Autodesk Inventor part; units mm, degrees
(part 2 of 2)
  line L767 (227.5411, -183.5124) -> (230.4279, -188.5124)
  line L768 (221.7676, -183.5124) -> (227.5411, -183.5124)
  line L769 (221.7676, -208.5124) -> (218.8809, -203.5124)
  line L770 (218.8809, -203.5124) -> (221.7676, -198.5124)
  line L771 (221.7676, -193.5124) -> (218.8809, -188.5124)
  line L772 (218.8809, -188.5124) -> (221.7676, -183.5124)
  line L773 (217.4375, -211.0124) -> (214.5507, -216.0124)
  line L774 (214.5507, -221.0124) -> (217.4375, -226.0124)
  line L775 (217.4375, -226.0124) -> (214.5507, -231.0124)
  line L776 (208.7772, -221.0124) -> (214.5507, -221.0124)
  line L777 (214.5507, -231.0124) -> (208.7772, -231.0124)
  line L778 (208.7772, -231.0124) -> (205.8905, -226.0124)
  line L779 (205.8905, -226.0124) -> (208.7772, -221.0124)
  line L780 (214.5507, -206.0124) -> (217.4375, -211.0124)
  line L781 (214.5507, -216.0124) -> (208.7772, -216.0124)
  line L782 (208.7772, -216.0124) -> (205.8905, -211.0124)
  line L783 (208.7772, -206.0124) -> (214.5507, -206.0124)
  line L784 (205.8905, -211.0124) -> (208.7772, -206.0124)
  line L785 (218.8809, -218.5124) -> (221.7676, -213.5124)
  line L786 (221.7676, -213.5124) -> (227.5411, -213.5124)
  line L787 (227.5411, -213.5124) -> (230.4279, -218.5124)
  line L788 (227.5411, -223.5124) -> (221.7676, -223.5124)
  line L789 (230.4279, -218.5124) -> (227.5411, -223.5124)
  line L790 (221.7676, -223.5124) -> (218.8809, -218.5124)
  line L791 (217.4375, -181.0124) -> (214.5507, -186.0124)
  line L792 (208.7772, -186.0124) -> (205.8905, -181.0124)
  line L793 (214.5507, -186.0124) -> (208.7772, -186.0124)
  line L794 (214.5507, -191.0124) -> (217.4375, -196.0124)
  line L795 (205.8905, -196.0124) -> (208.7772, -191.0124)
  line L796 (217.4375, -196.0124) -> (214.5507, -201.0124)
  line L797 (208.7772, -201.0124) -> (205.8905, -196.0124)
  line L798 (214.5507, -201.0124) -> (208.7772, -201.0124)
  line L799 (208.7772, -191.0124) -> (214.5507, -191.0124)
  line L800 (230.4279, -203.5124) -> (227.5411, -208.5124)
  line L801 (227.5411, -198.5124) -> (230.4279, -203.5124)
  point P0 (0, 0)
  point P1 (-256.336, -226.0124)
  point P2 (-243.3456, -218.5124)
  point P3 (-256.336, -211.0124)
  point P4 (-243.3456, -203.5124)
  point P5 (-256.336, -196.0124)
  point P6 (-243.3456, -188.5124)
  point P7 (-256.336, -181.0124)
  point P8 (-217.3456, -203.5124)
  point P9 (-217.3456, -188.5124)
  point P10 (-230.336, -226.0124)
  point P11 (-230.336, -211.0124)
  point P12 (-217.3456, -218.5124)
  point P13 (-230.336, -181.0124)
  point P14 (-230.336, -196.0124)
  point P15 (-191.3456, -203.5124)
  point P16 (-191.3456, -188.5124)
  point P17 (-204.336, -226.0124)
  point P18 (-204.336, -211.0124)
  point P19 (-191.3456, -218.5124)
  point P20 (-204.336, -181.0124)
  point P21 (-204.336, -196.0124)
  point P22 (-165.3456, -203.5124)
  point P23 (-165.3456, -188.5124)
  point P24 (-178.336, -226.0124)
  point P25 (-178.336, -211.0124)
  point P26 (-165.3456, -218.5124)
  point P27 (-178.336, -181.0124)
  point P28 (-178.336, -196.0124)
  point P29 (-139.3456, -203.5124)
  point P30 (-139.3456, -188.5124)
  point P31 (-152.336, -226.0124)
  point P32 (-152.336, -211.0124)
  point P33 (-139.3456, -218.5124)
  point P34 (-152.336, -181.0124)
  point P35 (-152.336, -196.0124)
  point P36 (-113.3456, -203.5124)
  point P37 (-113.3456, -188.5124)
  point P38 (-126.336, -226.0124)
  point P39 (-126.336, -211.0124)
  point P40 (-113.3456, -218.5124)
  point P41 (-126.336, -181.0124)
  point P42 (-126.336, -196.0124)
  point P43 (-87.3456, -203.5124)
  point P44 (-87.3456, -188.5124)
  point P45 (-100.336, -226.0124)
  point P46 (-100.336, -211.0124)
  point P47 (-87.3456, -218.5124)
  point P48 (-100.336, -181.0124)
  point P49 (-100.336, -196.0124)
  point P50 (-61.3456, -203.5124)
  point P51 (-61.3456, -188.5124)
  point P52 (-74.336, -226.0124)
  point P53 (-74.336, -211.0124)
  point P54 (-61.3456, -218.5124)
  point P55 (-74.336, -181.0124)
  point P56 (-74.336, -196.0124)
  point P57 (-35.3456, -203.5124)
  point P58 (-35.3456, -188.5124)
  point P59 (-48.336, -226.0124)
  point P60 (-48.336, -211.0124)
  point P61 (-35.3456, -218.5124)
  point P62 (-48.336, -181.0124)
  point P63 (-48.336, -196.0124)
  point P64 (-9.3456, -203.5124)
  point P65 (-9.3456, -188.5124)
  point P66 (-22.336, -226.0124)
  point P67 (-22.336, -211.0124)
  point P68 (-9.3456, -218.5124)
  point P69 (-22.336, -181.0124)
  point P70 (-22.336, -196.0124)
  point P71 (16.6544, -203.5124)
  point P72 (16.6544, -188.5124)
  point P73 (3.664, -226.0124)
  point P74 (3.664, -211.0124)
  point P75 (16.6544, -218.5124)
  point P76 (3.664, -181.0124)
  point P77 (3.664, -196.0124)
  point P78 (42.6544, -203.5124)
  point P79 (42.6544, -188.5124)
  point P80 (29.664, -226.0124)
  point P81 (29.664, -211.0124)
  point P82 (42.6544, -218.5124)
  point P83 (29.664, -181.0124)
  point P84 (29.664, -196.0124)
  point P85 (68.6544, -203.5124)
  point P86 (68.6544, -188.5124)
  point P87 (55.664, -226.0124)
  point P88 (55.664, -211.0124)
  point P89 (68.6544, -218.5124)
  point P90 (55.664, -181.0124)
  point P91 (55.664, -196.0124)
  point P92 (94.6544, -203.5124)
  point P93 (94.6544, -188.5124)
  point P94 (81.664, -226.0124)
  point P95 (81.664, -211.0124)
  point P96 (94.6544, -218.5124)
  point P97 (81.664, -181.0124)
  point P98 (81.664, -196.0124)
  point P99 (120.6544, -203.5124)
  point P100 (120.6544, -188.5124)
  point P101 (107.664, -226.0124)
  point P102 (107.664, -211.0124)
  point P103 (120.6544, -218.5124)
  point P104 (107.664, -181.0124)
  point P105 (107.664, -196.0124)
  point P106 (146.6544, -203.5124)
  point P107 (146.6544, -188.5124)
  point P108 (133.664, -226.0124)
  point P109 (133.664, -211.0124)
  point P110 (146.6544, -218.5124)
  point P111 (133.664, -181.0124)
  point P112 (133.664, -196.0124)
  point P113 (172.6544, -203.5124)
  point P114 (172.6544, -188.5124)
  point P115 (159.664, -226.0124)
  point P116 (159.664, -211.0124)
  point P117 (172.6544, -218.5124)
  point P118 (159.664, -181.0124)
  point P119 (159.664, -196.0124)
  point P120 (198.6544, -203.5124)
  point P121 (198.6544, -188.5124)
  point P122 (185.664, -226.0124)
  point P123 (185.664, -211.0124)
  point P124 (198.6544, -218.5124)
  point P125 (185.664, -181.0124)
  point P126 (185.664, -196.0124)
  point P127 (224.6544, -203.5124)
  point P128 (224.6544, -188.5124)
  point P129 (211.664, -226.0124)
  point P130 (211.664, -211.0124)
  point P131 (224.6544, -218.5124)
  point P132 (211.664, -181.0124)
  point P133 (211.664, -196.0124)
  dimension "d39" = 10
  dimension "d40" = 22
  dimension "d41" = 5
  dimension "d42" = 5
  dimension "d43" = 5
  dimension "d46" = 15
  dimension "d53" = 26
  constraints: 1596 end point, 4 horizontal, 2 parallel, 2 vertical alignment, 1 vertical, 1729 other
  measures "d39" distance between parallel lines of L5 L8
  measures "d40" distance between parallel lines of L2 L5
  measures "d41" distance between parallel lines of L10 L9
  measures "d42" distance between parallel lines of L8 L16
  measures "d43" distance between parallel lines of L21 L11
  measures "d46" distance of L10.end L23.start
  measures "d53" distance of L38.start L46.start
extrude "Extrusion2" cut sketch "Sketch4" against normal through all contours L4 L5 L6 L7 L8 L9 | L10 L11 L12 L13 L14 L15 | L16 L17 L18 L19 L20 L21 | L22 L24 L31 L32 L33 L23 | L25 L27 L30 L29 L28 L26 | L34 L36 L43 L44 L45 L35 | L37 L39 L42 L41 L40 L38 | L46 L77 L79 L78 L48 L47 | L49 L55 L56 L50 L87 L86 | L51 L52 L57 L58 L54 L53 | L59 L67 L68 L70 L69 L66 | L60 L61 L63 L64 L65 L62 | L71 L72 L73 L75 L74 L76 | L80 L82 L84 L83 L81 L85 | L88 L119 L121 L120 L90 L89 | L91 L97 L98 L92 L129 L128 | L93 L94 L99 L100 L96 L95 | L101 L109 L110 L112 L111 L108 | L102 L103 L105 L106 L107 L104 | L113 L114 L115 L117 L116 L118 | L122 L124 L126 L125 L123 L127 | L130 L161 L163 L162 L132 L131 | L133 L139 L140 L134 L171 L170 | L135 L136 L141 L142 L138 L137 | L143 L151 L152 L154 L153 L150 | L144 L145 L147 L148 L149 L146 | L155 L156 L157 L159 L158 L160 | L164 L166 L168 L167 L165 L169 | L172 L203 L205 L204 L174 L173 | L175 L181 L182 L176 L213 L212 | L177 L178 L183 L184 L180 L179 | L185 L193 L194 L196 L195 L192 | L186 L187 L189 L190 L191 L188 | L197 L198 L199 L201 L200 L202 | L206 L208 L210 L209 L207 L211 | L214 L245 L247 L246 L216 L215 | L217 L223 L224 L218 L255 L254 | L219 L220 L225 L226 L222 L221 | L227 L235 L236 L238 L237 L234 | L228 L229 L231 L232 L233 L230 | L239 L240 L241 L243 L242 L244 | L248 L250 L252 L251 L249 L253 | L256 L287 L289 L288 L258 L257 | L259 L265 L266 L260 L297 L296 | L261 L262 L267 L268 L264 L263 | L269 L277 L278 L280 L279 L276 | L270 L271 L273 L274 L275 L272 | L281 L282 L283 L285 L284 L286 | L290 L292 L294 L293 L291 L295 | L298 L329 L331 L330 L300 L299 | L301 L307 L308 L302 L339 L338 | L303 L304 L309 L310 L306 L305 | L311 L319 L320 L322 L321 L318 | L312 L313 L315 L316 L317 L314 | L323 L324 L325 L327 L326 L328 | L332 L334 L336 L335 L333 L337 | L340 L371 L373 L372 L342 L341 | L343 L349 L350 L344 L381 L380 | L345 L346 L351 L352 L348 L347 | L353 L361 L362 L364 L363 L360 | L354 L355 L357 L358 L359 L356 | L365 L366 L367 L369 L368 L370 | L374 L376 L378 L377 L375 L379 | L382 L413 L415 L414 L384 L383 | L385 L391 L392 L386 L423 L422 | L387 L388 L393 L394 L390 L389 | L395 L403 L404 L406 L405 L402 | L396 L397 L399 L400 L401 L398 | L407 L408 L409 L411 L410 L412 | L416 L418 L420 L419 L417 L421 | L424 L455 L457 L456 L426 L425 | L427 L433 L434 L428 L465 L464 | L429 L430 L435 L436 L432 L431 | L437 L445 L446 L448 L447 L444 | L438 L439 L441 L442 L443 L440 | L449 L450 L451 L453 L452 L454 | L458 L460 L462 L461 L459 L463 | L466 L497 L499 L498 L468 L467 | L469 L475 L476 L470 L507 L506 | L471 L472 L477 L478 L474 L473 | L479 L487 L488 L490 L489 L486 | L480 L481 L483 L484 L485 L482 | L491 L492 L493 L495 L494 L496 | L500 L502 L504 L503 L501 L505 | L508 L539 L541 L540 L510 L509 | L511 L517 L518 L512 L549 L548 | L513 L514 L519 L520 L516 L515 | L521 L529 L530 L532 L531 L528 | L522 L523 L525 L526 L527 L524 | L533 L534 L535 L537 L536 L538 | L542 L544 L546 L545 L543 L547 | L550 L581 L583 L582 L552 L551 | L553 L559 L560 L554 L591 L590 | L555 L556 L561 L562 L558 L557 | L563 L571 L572 L574 L573 L570 | L564 L565 L567 L568 L569 L566 | L575 L576 L577 L579 L578 L580 | L584 L586 L588 L587 L585 L589 | L592 L623 L625 L624 L594 L593 | L595 L601 L602 L596 L633 L632 | L597 L598 L603 L604 L600 L599 | L605 L613 L614 L616 L615 L612 | L606 L607 L609 L610 L611 L608 | L617 L618 L619 L621 L620 L622 | L626 L628 L630 L629 L627 L631 | L634 L665 L667 L666 L636 L635 | L637 L643 L644 L638 L675 L674 | L639 L640 L645 L646 L642 L641 | L647 L655 L656 L658 L657 L654 | L648 L649 L651 L652 L653 L650 | L659 L660 L661 L663 L662 L664 | L668 L670 L672 L671 L669 L673 | L676 L707 L709 L708 L678 L677 | L679 L685 L686 L680 L717 L716 | L681 L682 L687 L688 L684 L683 | L689 L697 L698 L700 L699 L696 | L690 L691 L693 L694 L695 L692 | L701 L702 L703 L705 L704 L706 | L710 L712 L714 L713 L711 L715 | L718 L749 L751 L750 L720 L719 | L721 L727 L728 L722 L759 L758 | L723 L724 L729 L730 L726 L725 | L731 L739 L740 L742 L741 L738 | L732 L733 L735 L736 L737 L734 | L743 L744 L745 L747 L746 L748 | L752 L754 L756 L755 L753 L757 | L760 L791 L793 L792 L762 L761 | L773 L781 L782 L784 L783 L780 | L774 L775 L777 L778 L779 L776 | L794 L796 L798 L797 L795 L799
equation "\"d2\" = d1"
equation "\"d8\" = d7"
equation "\"d10\" = d9"
equation "\"d11\" = d4"
equation "\"d42\" = d41"
equation "\"d43\" = d41"
equation "\"d9\" = d4"
body "Solid1"
